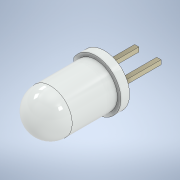
# Autodesk Inventor part: LED
Saved by Autodesk Inventor 2022 (Build 260153000, 153)
## iProperties
Created: 2024-06-27
Part Number: LED
Material: 一般
Document SubType Name: Modeling
Designer: yamashita1
Density: 1 g/cm^3
Appearance: 既定
Author: yamashita1
Autodesk Inventor part; units mm, degrees
ref_plane "YZ Plane" through (0, 0, 0) normal (1, 0, 0) x (0, 1, 0)
ref_plane "XZ Plane" through (0, 0, 0) normal (0, 1, 0) x (-1, 0, 0)
ref_plane "XY Plane" through (0, 0, 0) normal (0, 0, 1) x (1, 0, 0)
sketch "スケッチ1" plane through (0, 0, 0) normal (0, 0, 1) x (1, 0, 0)
  circle A0 centre (0, 0) radius 2.5
  dimension "d0" = 5
  constraints: 1 centre point, 1 coincident
  measures "d0" diameter of A0
extrude "押し出し1" add sketch "スケッチ1" along normal blind 7.7
fillet "フィレット1" radius 2.5 1 edges at (-2.5, 0, 7.7)
sketch "スケッチ2" plane through (0, 0, 0) normal (0, 0, -1) x (-1, 0, 0)
  circle A0 centre (0, 0) radius 2.9
  line L0 (2.5, 1.4697) -> (2.5, -1.4697)
  circle A1 centre (0, 0) radius 2.5 projected
  dimension "d4" = 5.8
  constraints: 2 end point, 2 point on circle, 1 centre point, 1 coincident, 1 tangent, 1 vertical
  measures "d4" diameter of A0
extrude "押し出し2" add sketch "スケッチ2" along normal blind 1 contours A1 | L0 A0 picked at (2.1443, -1.7224)
sketch "スケッチ3" plane through (0, 0, -1) normal (0, 0, -1) x (-1, 0, 0)
  line L0 (-1.52, 0.25) -> (-1.02, 0.25)
  line L1 (-1.02, 0.25) -> (-1.02, -0.25)
  line L2 (-1.02, -0.25) -> (-1.52, -0.25)
  line L3 (-1.52, -0.25) -> (-1.52, 0.25)
  line L4 (1.02, 0.25) -> (1.52, 0.25)
  line L5 (1.52, 0.25) -> (1.52, -0.25)
  line L6 (1.52, -0.25) -> (1.02, -0.25)
  line L7 (1.02, -0.25) -> (1.02, 0.25)
  line L8 (0, 1.603) -> (0, -1.603) construction
  line L9 (-1.27, -1.601) -> (-1.27, 1.6049) construction
  line L10 (1.27, 1.6049) -> (1.27, -1.601) construction
  point P0 (0, 0)
  point P1 (-1.02, 0)
  point P2 (1.02, 0)
  point P3 (0, 0)
  point P4 (-1.27, 0.25)
  point P5 (1.27, 0.25)
  dimension "d7" = 0.5
  dimension "d8" = 0.5
  dimension "d9" = 2.54
  constraints: 22 end point, 5 midpoint, 4 parallel, 3 point on line, 2 equal length, 2 horizontal, 2 horizontal alignment, 2 perpendicular, 1 coincident, 1 vertical, 1 other
  measures "d7" distance of L1.end L2.end
  measures "d8" distance of L0.end L1.end
  measures "d9" distance between parallel lines of L10 L9
extrude "押し出し3" add sketch "スケッチ3" along normal blind 5
